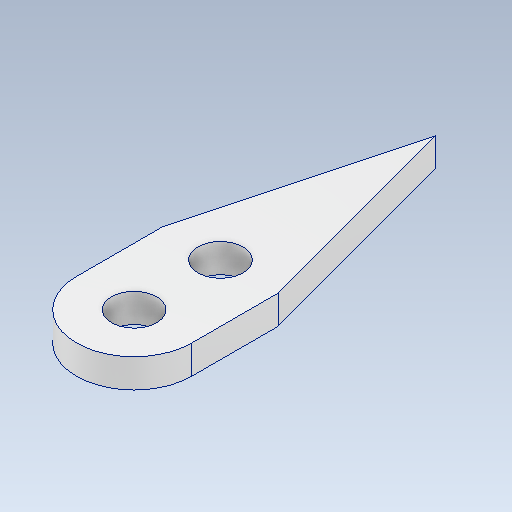
# Autodesk Inventor part: lock ring 2 supp
Saved by Autodesk Inventor 2021 (Build 250183000, 183)
## iProperties
Created: 2021-03-30
Part Number: lock ring 2 supp
Material: Aluminum 6061
Document SubType Name: Modeling
Designer: Work
Mass: 2.53626 g
Surface Area: 9.70651 cm^2
Volume: 0.939356 cm^3
Density: 2.7 g/cm^3
Appearance: Aluminum - Flat
Author: Work
Autodesk Inventor part; units mm, degrees
ref_plane "YZ Plane" through (0, 0, 0) normal (1, 0, 0) x (0, 1, 0)
ref_plane "XZ Plane" through (0, 0, 0) normal (0, 1, 0) x (-1, 0, 0)
ref_plane "XY Plane" through (0, 0, 0) normal (0, 0, 1) x (1, 0, 0)
sketch "Sketch1" plane through (0, 0, 0) normal (0, 1, 0) x (-1, 0, 0)
  line L0 (0, 0) -> (0, -9.525)
  arc A0 (6.35, 0) -> (-6.35, 0) centre (0, 0) ccw
  line L1 (6.35, 0) -> (6.35, -9.525)
  line L2 (-6.35, 0) -> (-6.35, -9.525)
  line L3 (6.35, -9.525) -> (0, -33.2235)
  line L4 (0, -33.2235) -> (-6.35, -9.525)
  dimension "d0" = 9.525
  dimension "d1" = 12.7
  dimension "d13" = 165
  dimension "d14" = 9.525
  dimension "d15" = 9.525
  dimension "d16" = 165
  constraints: 10 end point, 3 coincident, 3 vertical, 2 point on circle, 2 tangent, 1 centre point
  measures "d0" distance of L0.start L0.end
  measures "d1" diameter of A0
  measures "d13" angle of L1 L3
  measures "d14" distance of L2.start L2.end
  measures "d15" distance of L1.start L1.end
  measures "d16" angle of L2 L4
extrude "Extrusion1" add sketch "Sketch1" along normal blind 3.175
hole "Hole1" at (0, 0, 0) at (0, 0, -9.525) direction (0, 1, 0) diameter 4.9784 end through all clearance for "Flat Head Machine Screw (82)" size "#10" standard "Ansi Unified Screw Threads"
equation "\"d1\" = thickness"
equation "\"height\" = 203.2"
equation "\"thickness\" = 12.7"
equation "\"shaftDiam\" = 6.35"
equation "\"shaftSpace\" = 1.5875"
equation "\"stageSpace\" = 2.54"
equation "\"stageAngle\" = 15deg"
equation "\"bearingDiam\" = 9.5504"
equation "\"FlangeDiam\" = 12.7"
equation "\"FlangeDepth\" = 1.5875"
equation "\"smallFilet\" = 0.39687"
equation "\"ringDiam\" = 96.46608"
equation "\"stockHeight\" = 50.8"
equation "\"stockWidth\" = 76.2"
equation "\"stockRad\" = 9.525"
equation "\"stockGuage\" = 3.175"
equation "\"groundActu\" = 304.8"
equation "\"baseWidth\" = 1066.8"
equation "\"baseDepth\" = 254"
equation "\"capThickness\" = 3.175"
equation "\"sup1Len\" = 660.4"
equation "\"sup1Ang\" = 22.619865deg"
equation "\"sup2Len\" = 2079.37366"
equation "\"sup2Ang\" = 8.959949deg"
equation "\"supVertLen\" = 955.13561"
equation "\"supSideLen\" = 1531.12879"
equation "\"supSideAng\" = 19.376933deg"
body "Solid1"
